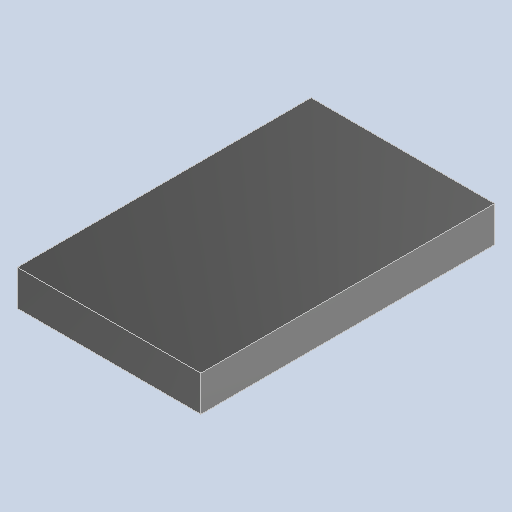
# Autodesk Inventor part: DK-42688-P_UpperCover
Saved by Autodesk Inventor 2024.2 (Build 282272000, 272)
## iProperties
Created: 2024-02-11
Part Number: DK-42688-P_UpperCover
Material: Acetal Resin, Black
Document SubType Name: Modeling
Designer: Masato Kubotera
Density: 1.425 g/cm^3
Appearance: Smooth - Black
Vendor: meviy
Author: Masato Kubotera
Autodesk Inventor part; units mm, degrees
ref_plane "YZ Plane" through (0, 0, 0) normal (1, 0, 0) x (0, 1, 0)
ref_plane "XZ Plane" through (0, 0, 0) normal (0, 1, 0) x (-1, 0, 0)
ref_plane "XY Plane" through (0, 0, 0) normal (0, 0, 1) x (1, 0, 0)
derived "DK-42688-P_Cover.ipt"
sketch "Sketch3" plane through (0, 0, 0) normal (0, 0, 1) x (1, 0, 0)
  line L0 (-34.55, 25.781) -> (48, 25.781) projected
  line L1 (-34.55, -25.781) -> (-34.55, 25.781) projected
  line L2 (48, -25.781) -> (-34.55, -25.781) projected
  line L3 (48, 25.781) -> (48, -25.781) projected
  line L4 (-34.55, 0) -> (48, 0) construction
  line L5 (6.725, -25.781) -> (6.725, 25.781) construction
  line L6 (43, 23.781) -> (-34.55, 23.781)
  line L7 (-34.55, -23.781) -> (43, -23.781)
  line L8 (43, -23.781) -> (43, 23.781)
  line L9 (-0.55, -25.781) -> (-0.55, -23.781)
  line L10 (10, -25.781) -> (10, -23.781)
  point P0 (0, 0)
  point P1 (6.725, 0)
  dimension "d1" = 2
  dimension "d2" = 5
  dimension "d3" = 34
  dimension "d4" = 38
  constraints: 14 end point, 6 point on line, 5 midpoint, 2 vertical, 1 horizontal, 1 parallel, 1 other
  measures "d1" distance between parallel lines of L0 L6
  measures "d2" distance between parallel lines of L3 L8
  measures "d3" distance between parallel lines of L1 L9
  measures "d4" distance between parallel lines of L3 L10
extrude "Extrusion1" add sketch "Sketch3" against normal blind 1
extrude "Extrusion2" add sketch "Sketch3" against normal blind 10 contours L0 L3 L2 L10 L7 L8 L6 L1 | L7 L9 L2 L1
fillet "Fillet1" radius 1.5 2 edges at (43, -23.781, -5.5) (43, 23.781, -5.5)
extrude "Extrusion3" add sketch "Sketch3" against normal blind 7 contours L2 L9 L7 L10
sketch "Sketch2" plane through (0, 0, 0) normal (0, 0, 1) x (1, 0, 0)
  line L0 (-50, 0) -> (50, 0) construction
  line L1 (-34.55, 25.781) -> (48, 25.781) construction
  line L2 (48, 25.781) -> (48, -25.781) construction
  line L3 (48, -25.781) -> (-34.55, -25.781) construction
  line L4 (-34.55, -25.781) -> (-34.55, 25.781) construction
  line L5 (-34.55, 25.781) -> (48, -25.781) construction
  line L6 (48, 25.781) -> (-34.55, -25.781) construction
  line L7 (-35.05, -26.281) -> (48.5, -26.281) projected
  line L8 (48.5, -26.281) -> (48.5, 26.281) projected
  line L9 (48.5, 26.281) -> (-35.05, 26.281) projected
  line L10 (-35.05, 26.281) -> (-35.05, -26.281) projected
  line L11 (-35.05, -26.281) -> (48.5, 26.281) construction
  line L12 (48.5, -26.281) -> (-35.05, 26.281) construction
  line L13 (6.725, 25.781) -> (6.725, -25.781) construction
  line L14 (-35.05, -24.781) -> (-50, -24.781) projected
  circle A0 centre (-47, 29.5) radius 3 construction
  circle A1 centre (-47, 29.5) radius 1.6 construction
  circle A2 centre (47, 29.5) radius 3 construction
  circle A3 centre (47, 29.5) radius 1.6 construction
  line L15 (50, -32.5) -> (50, 32.5) projected
  line L16 (50, 32.5) -> (-50, 32.5) projected
  line L17 (-50, -32.5) -> (50, -32.5) projected
  line L18 (-50, 32.5) -> (-50, -32.5) projected
  line L19 (-34.05, 25.281) -> (-34.05, -25.281) projected
  line L20 (47.5, -23.281) -> (47.5, 23.281) projected
  arc A4 (45.5, -25.281) -> (47.5, -23.281) centre (45.5, -23.281) ccw projected
  arc A5 (47.5, 23.281) -> (45.5, 25.281) centre (45.5, 23.281) ccw projected
  line L21 (13, 23.281) -> (13, -23.281) projected
  line L22 (10, -23.281) -> (10, 23.281) projected
  line L23 (45.5, 25.281) -> (15, 25.281) projected
  line L24 (8, 25.281) -> (-34.05, 25.281) projected
  line L25 (-34.05, -25.281) -> (8, -25.281) projected
  line L26 (15, -25.281) -> (45.5, -25.281) projected
  arc A6 (13, -23.281) -> (15, -25.281) centre (15, -23.281) ccw projected
  arc A7 (15, 25.281) -> (13, 23.281) centre (15, 23.281) ccw projected
  arc A8 (10, 23.281) -> (8, 25.281) centre (8, 23.281) ccw projected
  arc A9 (8, -25.281) -> (10, -23.281) centre (8, -23.281) ccw projected
  arc A10 (46.3787, -26.281) -> (48.5, -24.1597) centre (47.4393, -25.2203) ccw projected
  arc A11 (48.5, 24.1597) -> (46.3787, 26.281) centre (47.4393, 25.2203) ccw projected
  line L27 (-35.05, 24.781) -> (-50, 24.781) projected
  arc A12 (-32.05, 26.281) -> (-35.05, 26.281) centre (-33.55, 26.281) ccw projected
  arc A13 (-35.05, -26.281) -> (-32.05, -26.281) centre (-33.55, -26.281) ccw projected
  line L28 (40, 32.5) -> (36.5, 29) projected
  line L29 (36.5, 29) -> (-36.5, 29) projected
  line L30 (-36.5, 29) -> (-40, 32.5) projected
  line L31 (0, -126) -> (0, 126) projected
  line L32 (40, -32.5) -> (36.5, -29) projected
  line L33 (36.5, -29) -> (-36.5, -29) projected
  line L34 (-36.5, -29) -> (-40, -32.5) projected
  arc A14 (-34.05, -22.4526) -> (-31.2216, -25.281) centre (-32.6358, -23.8668) ccw projected
  arc A15 (-31.2216, 25.281) -> (-34.05, 22.4526) centre (-32.6358, 23.8668) ccw projected
  point P0 (6.725, 0)
  point P1 (0, 0)
  point P2 (6.725, 0)
  point P3 (-47, -29.5)
  point P4 (47, -29.5)
  constraints: 2 other
body "Solid1"
